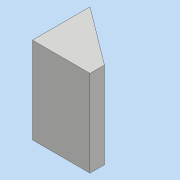
# Autodesk Inventor part: 9
Saved by Autodesk Inventor 2017 (Build 210142000, 142)
## iProperties
Part Number: 9
Material: 一般
Document SubType Name: Modeling
Designer: d8910
Density: 1 g/cm^3
Appearance: 預設
Author: d8910
Autodesk Inventor part; units mm, degrees
ref_plane "YZ Plane" through (0, 0, 0) normal (1, 0, 0) x (0, 1, 0)
ref_plane "XZ Plane" through (0, 0, 0) normal (0, 1, 0) x (-1, 0, 0)
sketch "草圖1" plane through (0, 0, 0) normal (0, 1, 0) x (-1, 0, 0)
  line L0 (10, 15) -> (-10, 15)
  line L1 (-10, 15) -> (-10, -15)
  line L2 (-10, -15) -> (10, -15)
  line L3 (10, -15) -> (10, 15)
  point P0 (0, 0)
  point P1 (10, 0)
  point P2 (0, -15)
  dimension "d0" = 30
  dimension "d1" = 20
  constraints: 8 end point, 2 midpoint, 2 parallel, 1 horizontal, 1 horizontal alignment, 1 perpendicular, 1 vertical alignment
  measures "d0" distance of L2.end L0.start
  measures "d1" distance of L1.end L2.end
extrude "擠出1" add sketch "草圖1" along normal blind 5
sketch "草圖2" plane through (-10, 0, 15) normal (0, 0, 1) x (1, 0, 0)
  line L0 (0, 5) -> (20, 5) projected
  line L1 (0, 5) -> (0, 20)
  line L2 (0, 20) -> (20, 5)
  line L3 (20, 5) -> (0, 5)
  point P0 (10, 0)
  dimension "d4" = 15
  constraints: 6 end point, 1 perpendicular, 1 vertical
  measures "d4" distance of L0.start L1.end
extrude "擠出2" add sketch "草圖2" against normal blind 10
mirror "鏡射1" about plane through (0, 0, 0) normal (0, 0, 1) of "擠出2"
ref_plane "工作平面1" through (0, 28.75, 0) normal (0, 1, 0) x (1, 0, 0)
sketch "草圖3" plane through (0, 28.75, 0) normal (0, 1, 0) x (1, 0, 0)
  line L0 (10, 5) -> (-10, 5) construction
  line L1 (-10, 5) -> (-10, -5) construction
  line L2 (-10, -5) -> (10, -5) construction
  line L3 (10, -5) -> (10, 5) construction
  line L4 (10, -15) -> (-10, -15) construction
  line L5 (10, -15) -> (10, -5) construction
  line L6 (-10, -5) -> (10, -5) construction
  line L7 (-10, -15) -> (-10, -5) construction
  line L8 (10, 15) -> (-10, 15) construction
  line L9 (-10, 15) -> (-10, 5) construction
  line L10 (-10, 5) -> (10, 5) construction
  line L11 (10, 5) -> (10, 15) construction
  line L12 (-10, -5) -> (10, -10) construction
  line L13 (10, -15) -> (10, 15) construction
  line L14 (10, -10) -> (10, 10) construction
  line L15 (-10, 5) -> (10, 10) construction
  line L16 (-10, 5) -> (-10, -5) construction
  line L17 (-10, -5) -> (-10, 5)
  line L18 (10, 10) -> (-10, 5)
  line L19 (-10, -5) -> (10, -10)
  line L20 (10, -10) -> (10, 10)
  point P0 (0, 0)
  dimension "d8" = 10
  constraints: 16 end point, 2 collinear, 2 point on line, 1 midpoint, 1 perpendicular
  measures "d8" horizontal distance of point (0, 0) L14.end
extrude "擠出3" cut sketch "草圖3" against normal up to surface (23.75 mm away)
